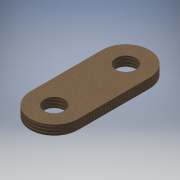
# Autodesk Inventor part: podstawa
Saved by Autodesk Inventor 2017 (Build 210142000, 142)
## iProperties
Created: 2017-03-24
Part Number: podstawa
Material: MDF - płyta pilśniowa o średniej gęstości
Document SubType Name: Modeling
Designer: Damian
Density: 0.8 g/cm^3
Appearance: Tektura - falista
Author: Damian
Autodesk Inventor part; units mm, degrees
ref_plane "YZ Plane" through (0, 0, 0) normal (1, 0, 0) x (0, 1, 0)
ref_plane "XZ Plane" through (0, 0, 0) normal (0, 1, 0) x (-1, 0, 0)
ref_plane "XY Plane" through (0, 0, 0) normal (0, 0, 1) x (1, 0, 0)
sketch "Szkic1" plane through (0, 0, 0) normal (0, 0, 1) x (1, 0, 0)
  line L0 (0, -75) -> (0, 75) construction
  line L1 (50, -75) -> (50, 75)
  line L2 (-50, 75) -> (-50, -75)
  arc A0 (-50, -75) -> (50, -75) centre (0, -75) ccw
  arc A1 (50, 75) -> (-50, 75) centre (0, 75) ccw
  point P0 (0, 0)
  dimension "d2" = 100
  constraints: 8 end point, 4 point on circle, 4 tangent, 2 centre point, 1 midpoint, 1 parallel, 1 vertical
  measures "d2" diameter of A1
extrude "Wyciągnięcie proste2" add sketch "Szkic1" along normal blind 20
sketch "Szkic2" plane through (0, 0, 20) normal (0, 0, 1) x (1, 0, 0)
  circle A0 centre (0, 75) radius 21.05
  circle A1 centre (0, -75) radius 21.05
  point P0 (0, 0)
  dimension "d7" = 42.1
  dimension "d8" = 42.1
  constraints: 2 centre point
  measures "d7" diameter of A0
  measures "d8" diameter of A1
extrude "Wyciągnięcie proste3" cut sketch "Szkic2" against normal blind 12
sketch "Szkic3" plane through (0, -75, 8) normal (0, 0, 1) x (1, 0, 0)
  circle A0 centre (0, 0) radius 17.5
  point P0 (0, 75)
  dimension "d11" = 35
  constraints: 1 centre point
  measures "d11" diameter of A0
sketch "Szkic4" plane through (0, 75, 8) normal (0, 0, 1) x (1, 0, 0)
  circle A0 centre (0, 0) radius 17.5
  point P0 (0, -75)
  dimension "d12" = 35
  constraints: 1 centre point
  measures "d12" diameter of A0
extrude "Wyciągnięcie proste4" cut sketch "Szkic4" against normal blind 12
extrude "Wyciągnięcie proste5" cut sketch "Szkic3" against normal blind 12
equation "\"d12\" = d11"
